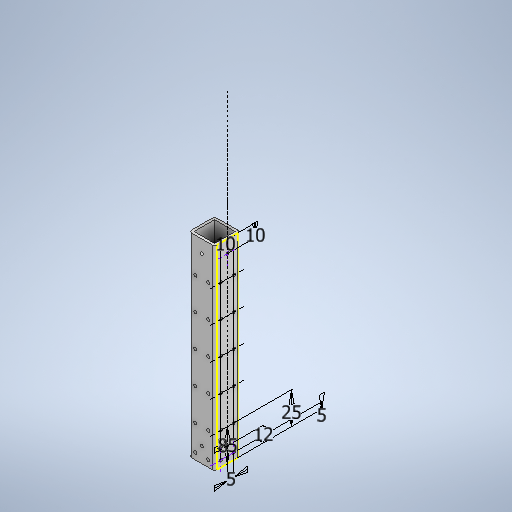
# Autodesk Inventor part: verticalaxle
Saved by Autodesk Inventor 2025.2 (Build 292293000, 293)
## iProperties
Created: 2026-03-22
Part Number: verticalaxle
Material: Generic
Document SubType Name: Modeling
Designer: hp
Density: 1 g/cm^3
Appearance: Default
Author: hp
Autodesk Inventor part; units mm, degrees
ref_plane "YZ Plane" through (0, 0, 0) normal (1, 0, 0) x (0, 1, 0)
ref_plane "XZ Plane" through (0, 0, 0) normal (0, 1, 0) x (-1, 0, 0)
ref_plane "XY Plane" through (0, 0, 0) normal (0, 0, 1) x (1, 0, 0)
sketch "Sketch1" plane through (0, 0, 0) normal (0, 1, 0) x (-1, 0, 0)
  line L0 (8, 10) -> (-8, 10)
  line L1 (-10, 8) -> (-10, -8)
  line L2 (-8, -10) -> (8, -10)
  line L3 (10, -8) -> (10, 8)
  line L4 (10, 10) -> (-10, -10) construction
  line L5 (-10, 10) -> (10, -10) construction
  line L6 (8, 8) -> (-8, 8)
  line L7 (-8, 8) -> (-8, -8)
  line L8 (-8, -8) -> (8, -8)
  line L9 (8, -8) -> (8, 8)
  arc A0 (10, 8) -> (8, 10) centre (8, 8) ccw
  arc A1 (8, -10) -> (10, -8) centre (8, -8) ccw
  arc A2 (-10, -8) -> (-8, -10) centre (-8, -8) ccw
  arc A3 (-8, 10) -> (-10, 8) centre (-8, 8) ccw
  point P0 (0, 0)
  dimension "d0" = 20
  dimension "d1" = 20
  dimension "d2" = 2
  dimension "d3" = 2
  constraints: 20 end point, 8 point on circle, 8 point on line, 8 tangent, 4 centre point, 4 parallel, 3 equal radius, 2 midpoint, 2 perpendicular, 1 horizontal, 3 other
  measures "d0" distance of L5.end L4.end
  measures "d1" distance of L4.end L5.start
  measures "d2" distance between parallel lines of L3 L9
  measures "d3" radius of A0
extrude "Extrusion1" add sketch "Sketch1" along normal blind 152
sketch "Sketch2" plane through (10, 0, 8) normal (1, 0, 0) x (0, 0, -1)
  line L0 (0, 0) -> (0, 152) projected
  line L1 (16, 0) -> (16, 152) projected
  line L2 (0, 0) -> (16, 0) projected
  line L3 (0, 152) -> (16, 152) projected
  line L4 (8, 0) -> (8, 152) construction
  line L5 (8, 25) -> (8, 177) construction
  line L6 (8, 50) -> (8, 202) construction
  line L7 (8, 75) -> (8, 227) construction
  line L8 (8, 100) -> (8, 252) construction
  point P0 (8, 12)
  point P1 (8, 142)
  point P2 (13, 25)
  point P3 (13, 50)
  point P4 (13, 75)
  point P5 (13, 100)
  point P6 (13, 125)
  point P7 (3, 25)
  point P8 (3, 50)
  point P9 (3, 75)
  point P10 (3, 100)
  point P11 (3, 125)
  point P12 (13, 5)
  point P13 (3, 5)
  dimension "d6" = 12
  dimension "d7" = 8
  dimension "d22" = 10
  dimension "d23" = 5
  dimension "d24" = 25
  dimension "d27" = 25
  dimension "d130" = 10
  dimension "d159" = 5
  constraints: 10 end point, 5 symmetric about line, 1 collinear, 1 midpoint, 1 vertical, 15 other
  measures "d6" distance from line of L2 point (8, 12)
  measures "d7" distance from line of point (8, 12) L0
  measures "d22" distance from line of point (8, 142) L3
  measures "d23" distance from line of L4 point (13, 25)
  measures "d24" distance from line of L2 point (13, 25)
  measures "d27" distance of L4.start L5.start
  measures "d130" distance of point (3, 5) point (13, 5)
  measures "d159" distance from line of L2 point (13, 5)
hole "Hole1" at (10, 12, 0) at (10, 142, 0) direction (-1, 0, 0) diameter 2.45 depth 2 tip angle 118
pattern_circular "Circular Pattern1" count 4 over 360 about axis through (0, -10, 0) along (0, 1, 0) of "Hole1"
thread "Thread1" size "M2.5x0.45" class "6H" standard "ANSI Metric M Profile" full length
thread "Thread2" size "M2.5x0.45" class "6H" standard "ANSI Metric M Profile" full length
hole "Hole2" at (10, 125, -5) at (10, 125, 5) at (10, 100, 5) at (10, 100, -5) at (10, 75, 5) at (10, 75, -5) at (10, 50, -5) at (10, 50, 5) at (10, 25, -5) at (10, 25, 5) direction (-1, 0, 0) diameter 2.45 depth 2 tip angle 118
thread "Thread3" size "M2.5x0.45" class "6H" standard "ISO Metric profile" length 8
thread "Thread4" size "M2.5x0.45" class "6H" standard "ISO Metric profile" length 8
thread "Thread5" size "M2.5x0.45" class "6H" standard "ISO Metric profile" length 8
thread "Thread6" size "M2.5x0.45" class "6H" standard "ISO Metric profile" length 8
thread "Thread7" size "M2.5x0.45" class "6H" standard "ISO Metric profile" length 8
thread "Thread8" size "M2.5x0.45" class "6H" standard "ISO Metric profile" length 8
thread "Thread9" size "M2.5x0.45" class "6H" standard "ISO Metric profile" length 8
thread "Thread10" size "M2.5x0.45" class "6H" standard "ISO Metric profile" length 8
thread "Thread11" size "M2.5x0.45" class "6H" standard "ISO Metric profile" length 8
thread "Thread12" size "M2.5x0.45" class "6H" standard "ISO Metric profile" length 8
thread "Thread13" size "M2.5x0.45" class "6H" standard "ISO Metric profile" length 8
pattern_circular "Circular Pattern2" count 4 over 360 about axis through (0, -10, 0) along (0, 1, 0) of "Hole2"
thread "Thread14" size "M2.5x0.45" class "6H" standard "ISO Metric profile" length 8
thread "Thread15" size "M2.5x0.45" class "6H" standard "ISO Metric profile" length 8
thread "Thread16" size "M2.5x0.45" class "6H" standard "ISO Metric profile" length 8
thread "Thread17" size "M2.5x0.45" class "6H" standard "ISO Metric profile" length 8
thread "Thread18" size "M2.5x0.45" class "6H" standard "ISO Metric profile" length 8
thread "Thread19" size "M2.5x0.45" class "6H" standard "ISO Metric profile" length 8
thread "Thread20" size "M2.5x0.45" class "6H" standard "ISO Metric profile" length 8
thread "Thread21" size "M2.5x0.45" class "6H" standard "ISO Metric profile" length 8
thread "Thread22" size "M2.5x0.45" class "6H" standard "ISO Metric profile" length 8
thread "Thread23" size "M2.5x0.45" class "6H" standard "ISO Metric profile" length 8
thread "Thread24" size "M2.5x0.45" class "6H" standard "ISO Metric profile" length 8
thread "Thread25" size "M2.5x0.45" class "6H" standard "ISO Metric profile" length 8
thread "Thread26" size "M2.5x0.45" class "6H" standard "ISO Metric profile" length 8
thread "Thread27" size "M2.5x0.45" class "6H" standard "ISO Metric profile" length 8
thread "Thread28" size "M2.5x0.45" class "6H" standard "ISO Metric profile" length 8
thread "Thread29" size "M2.5x0.45" class "6H" standard "ISO Metric profile" length 8
thread "Thread30" size "M2.5x0.45" class "6H" standard "ISO Metric profile" length 8
thread "Thread31" size "M2.5x0.45" class "6H" standard "ISO Metric profile" length 8
thread "Thread32" size "M2.5x0.45" class "6H" standard "ISO Metric profile" length 8
thread "Thread33" size "M2.5x0.45" class "6H" standard "ISO Metric profile" length 8
thread "Thread34" size "M2.5x0.45" class "6H" standard "ISO Metric profile" length 8
thread "Thread35" size "M2.5x0.45" class "6H" standard "ISO Metric profile" length 8
thread "Thread36" size "M2.5x0.45" class "6H" standard "ISO Metric profile" length 8
thread "Thread37" size "M2.5x0.45" class "6H" standard "ISO Metric profile" length 8
thread "Thread38" size "M2.5x0.45" class "6H" standard "ISO Metric profile" length 8
thread "Thread39" size "M2.5x0.45" class "6H" standard "ISO Metric profile" length 8
thread "Thread40" size "M2.5x0.45" class "6H" standard "ISO Metric profile" length 8
thread "Thread41" size "M2.5x0.45" class "6H" standard "ISO Metric profile" length 8
thread "Thread42" size "M2.5x0.45" class "6H" standard "ISO Metric profile" length 8
thread "Thread43" size "M2.5x0.45" class "6H" standard "ISO Metric profile" length 8
thread "Thread44" size "M2.5x0.45" class "6H" standard "ISO Metric profile" length 8
thread "Thread45" size "M2.5x0.45" class "6H" standard "ISO Metric profile" length 8
thread "Thread46" size "M2.5x0.45" class "6H" standard "ISO Metric profile" length 8
hole "Hole3" at (10, 5, -5) at (10, 5, 5) direction (-1, 0, 0) diameter 2.45 depth 2 tip angle 118
thread "Thread47" size "M2.5x0.45" class "6H" standard "ISO Metric profile" length 8
thread "Thread48" size "M2.5x0.45" class "6H" standard "ISO Metric profile" length 8
pattern_circular "Circular Pattern3" count 4 over 360 about axis through (0, -10, 0) along (0, 1, 0) of "Hole3"
thread "Thread49" size "M2.5x0.45" class "6H" standard "ISO Metric profile" length 8
thread "Thread50" size "M2.5x0.45" class "6H" standard "ISO Metric profile" length 8
thread "Thread51" size "M2.5x0.45" class "6H" standard "ISO Metric profile" length 9.967
thread "Thread52" size "M2.5x0.45" class "6H" standard "ISO Metric profile" length 9.967
thread "Thread53" size "M2.5x0.45" class "6H" standard "ISO Metric profile" length 9.967
thread "Thread54" size "M2.5x0.45" class "6H" standard "ISO Metric profile" length 9.967
body "Solid1"
